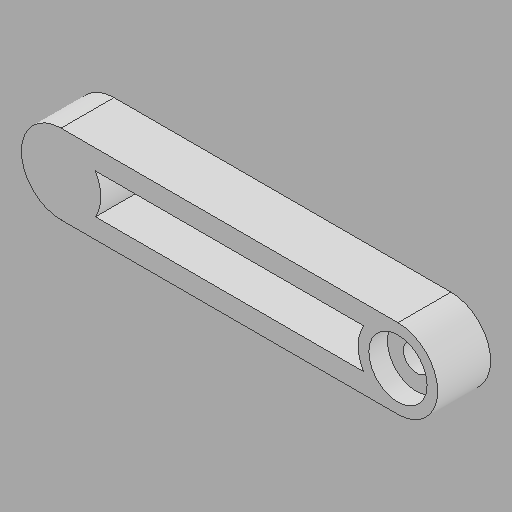
# Autodesk Inventor part: PARALLEL_LINKAGE_LH
Saved by Autodesk Inventor 2025.2 (Build 292293000, 293)
## iProperties
Created: 2026-06-03
Part Number: PARALLEL_LINKAGE_LH
Material: Generic
Document SubType Name: Modeling
Designer: Ben
Density: 1 g/cm^3
Appearance: Default
Author: Ben
Autodesk Inventor part; units mm, degrees
ref_plane "YZ Plane" through (0, 0, 0) normal (1, 0, 0) x (0, 1, 0)
ref_plane "XZ Plane" through (0, 0, 0) normal (0, 1, 0) x (-1, 0, 0)
ref_plane "XY Plane" through (0, 0, 0) normal (0, 0, 1) x (1, 0, 0)
sketch "Sketch1" plane through (0, 0, 0) normal (0, 0, 1) x (1, 0, 0)
  circle A0 centre (0, 0) radius 15
  circle A1 centre (127.2387, 0) radius 15
  line L0 (0, 15) -> (127.2387, 15)
  line L1 (0, -15) -> (127.2387, -15)
  line L2 (12.9904, -7.5) -> (114.2483, -7.5)
  line L3 (12.9904, 7.5) -> (114.2483, 7.5)
  dimension "d0" = 30
  dimension "d1" = 127.2387
  dimension "d2" = 7.5
  dimension "d3" = 7.5
  constraints: 8 end point, 8 point on circle, 3 tangent, 2 centre point, 2 parallel, 1 coincident, 1 equal radius, 1 horizontal, 1 horizontal alignment
  measures "d0" diameter of A0
  measures "d1" distance of A1.centre point (0, 0)
  measures "d2" distance between parallel lines of L1 L2
  measures "d3" distance between parallel lines of L0 L3
extrude "Extrusion1" add sketch "Sketch1" along normal blind 20 contours A0 | A0 L0 A1 L3 | L2 A1 L1 A0 | A1
sketch "Sketch2" plane through (0, 0, 20) normal (0, 0, 1) x (1, 0, 0)
  arc A0 (127.2387, -15) -> (127.2387, 15) centre (127.2387, 0) ccw projected
  point P0 (0, 0)
  point P1 (142.2387, 0)
  constraints: 1 coincident, 1 horizontal alignment, 1 point on circle
hole "Hole1" at (127.2387, 0, 20) direction (0, 0, -1) diameter 10 end through all counterbore diameter 22 counterbore depth 7
body "Solid1"
